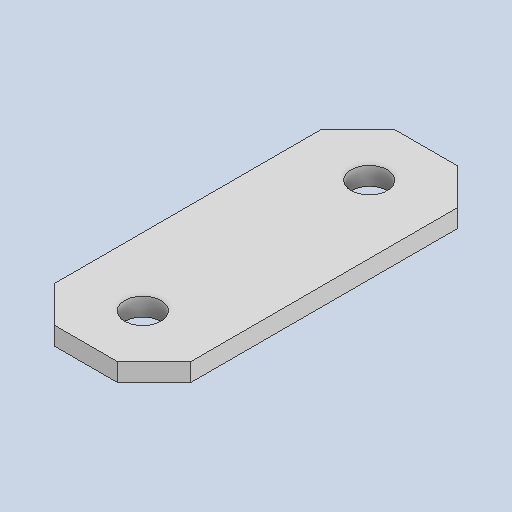
# Autodesk Inventor part: A1_joiners
Saved by Autodesk Inventor 2025.2 (Build 292293000, 293)
## iProperties
Created: 2025-03-24
Part Number: A1_joiners
Material: Generic
Document SubType Name: Sheet Metal
Designer: Caspe
Density: 1 g/cm^3
Sheet Metal Rule: Default_mm
Appearance: Default
Author: Caspe
Autodesk Inventor part; units mm, degrees
ref_plane "YZ Plane" through (0, 0, 0) normal (1, 0, 0) x (0, 1, 0)
ref_plane "XZ Plane" through (0, 0, 0) normal (0, 1, 0) x (-1, 0, 0)
ref_plane "XY Plane" through (0, 0, 0) normal (0, 0, 1) x (1, 0, 0)
sketch "Sketch1" plane through (0, 0, 0) normal (0, 1, 0) x (-1, 0, 0)
  line L0 (0, 0) -> (15, 0)
  line L1 (15, 0) -> (15, -37.5)
  line L2 (15, -37.5) -> (0, -37.5)
  line L3 (0, -37.5) -> (0, 0)
  line L4 (0, -18.75) -> (15, -18.75)
  circle A0 centre (7.5, -6.25) radius 2
  circle A1 centre (7.5, -31.25) radius 2
  dimension "d0" = 37.5
  dimension "d1" = 15
  dimension "d2" = 4
  dimension "d3" = 7.5
  dimension "d4" = 12.5
  measures "d0" distance of L0.end L1.end
  measures "d1" distance between parallel lines of L3 L1
  measures "d2" diameter of A0
  measures "d3" distance from line of L3 A0.centre
  measures "d4" distance from line of L4 A0.centre
extrude "Plate1" add sketch "Sketch1" along normal blind 2
chamfer "Corner Chamfer1" distance 4 angle 45 4 edges at (-15, 1, 0) (0, 1, 0) (-15, 1, -37.5) (0, 1, -37.5)
equation "\"d0\" = 0.75 * A_width"
equation "\"d2\" = rivet_diameter"
equation "\"d3\" = 0.5 * d1"
equation "\"d4\" = 0.25 * A_width"
equation "\"d5\" = Thickness"
equation "\"Thickness\" = plate_thickness"
equation "\"BendRadius\" = Thickness"
equation "\"BendReliefWidth\" = Thickness"
equation "\"BendReliefDepth\" = 0.5 * Thickness"
equation "\"CornerReliefSize\" = 4 * Thickness"
equation "\"MinimumRemnant\" = 2 * Thickness"
equation "\"TransitionRadius\" = BendRadius"
equation "\"JacobiRadiusSize\" = BendRadius"
equation "\"GapSize\" = Thickness"
equation "\"A_joint_tolerance\" = 3"
equation "\"l___________\" = 0"
equation "\"l__________\" = 0"
equation "\"l_________\" = 0"
equation "\"rivet_diameter\" = 4"
equation "\"plate_thickness\" = 2"
equation "\"l________\" = 0"
equation "\"A_B_spacing\" = 2"
equation "\"A_width\" = 50"
body "Solid1"
